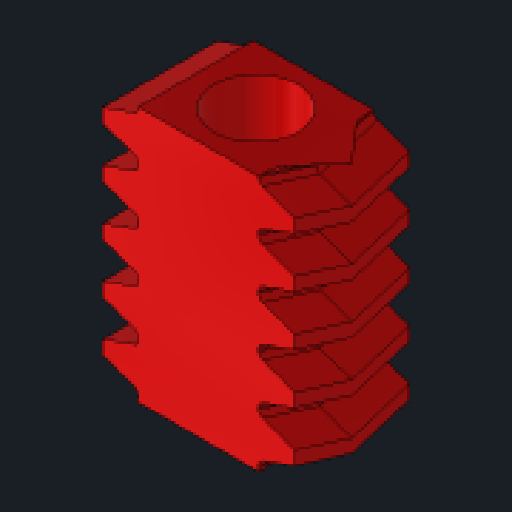
# Autodesk Inventor part: rack
Saved by Autodesk Inventor 2023.2 (Build 272271030, 271C)
## iProperties
Created: 2023-10-23
Part Number: rack
Material: Generic
Document SubType Name: Modeling
Designer: robpl
Density: 1 g/cm^3
Appearance: Red
Author: robpl
## iProperties of the stored document rack_3DPrint.ipt
Created: 2023-10-23
Part Number: rack_3DPrint
Material: Generic
Document SubType Name: Modeling
Designer: robpl
Density: 1 g/cm^3
Appearance: Default
Author: robpl
Autodesk Inventor part; units mm, degrees
ref_plane "YZ Plane" through (0, 0, 0) normal (1, 0, 0) x (0, 1, 0)
sketch "Sketch1" plane through (0, 0, 0) normal (0, 0, 1) x (1, 0, 0)
  line L0 (0, 0) -> (14.5, 0)
  line L1 (14.5, 0) -> (14.5, 20)
  line L2 (14.5, 20) -> (0, 20)
  line L3 (0, 20) -> (0, 0)
  dimension "d0" = 14.5
  dimension "d1" = 20
  constraints: 8 end point, 2 parallel, 1 horizontal, 1 perpendicular
  measures "d0" distance of L2.end L1.end
  measures "d1" distance of L1.end L0.end
extrude "Extrusion1" add sketch "Sketch1" along normal blind 4.5
sketch "Sketch2" plane through (0, 0, 4.5) normal (0, 0, 1) x (1, 0, 0)
  line L0 (14.5, 0) -> (14.5, 20) projected
  line L1 (14.5, 20) -> (0, 20) projected
  line L2 (0, 20) -> (0, 0) projected
  line L3 (0, 0) -> (14.5, 0) projected
  line L4 (14.5, 0) -> (14.5, 20) projected
  line L5 (14.5, 21.4367) -> (11.6875, 20.413)
  line L6 (11.6875, 20.413) -> (11.6875, 19.587)
  line L7 (11.6875, 19.587) -> (14.5, 18.5633)
  line L8 (14.5, 17.5097) -> (11.6875, 16.4861)
  line L9 (11.6875, 16.4861) -> (11.6875, 15.66)
  line L10 (11.6875, 15.66) -> (14.5, 14.6363)
  arc A0 (12, 20.5268) -> (11.6875, 20.0804) centre (12.1625, 20.0804) ccw
  arc A1 (11.6875, 19.9196) -> (12, 19.4732) centre (12.1625, 19.9196) ccw
  line L11 (14.5, 20) -> (0, 20) projected
  arc A2 (11.6875, 15.9926) -> (12, 15.5462) centre (12.1625, 15.9926) ccw
  arc A3 (12, 16.5998) -> (11.6875, 16.1535) centre (12.1625, 16.1535) ccw
  line L12 (14.5, 21.4367) -> (14.5, 18.5633)
  line L13 (7.25, 20) -> (7.25, 0)
  line L14 (0, 0) -> (14.5, 0) projected
  line L15 (0, 21.4367) -> (2.8125, 20.413)
  line L16 (2.8125, 20.413) -> (2.8125, 19.587)
  line L17 (2.8125, 19.587) -> (0, 18.5633)
  arc A4 (2.8125, 20.0804) -> (2.5, 20.5268) centre (2.3375, 20.0804) ccw
  arc A5 (2.5, 19.4732) -> (2.8125, 19.9196) centre (2.3375, 19.9196) ccw
  line L18 (0, 21.4367) -> (0, 18.5633)
  line L19 (0, 17.5097) -> (2.8125, 16.4861)
  line L20 (2.8125, 16.4861) -> (2.8125, 15.66)
  line L21 (2.8125, 15.66) -> (0, 14.6363)
  arc A6 (2.5, 15.5462) -> (2.8125, 15.9926) centre (2.3375, 15.9926) ccw
  arc A7 (2.8125, 16.1535) -> (2.5, 16.5998) centre (2.3375, 16.1535) ccw
  point P0 (11.6875, 20)
  point P1 (13.25, 19.0183)
  point P2 (13.25, 17.0548)
  point P3 (14.5, 18.5633)
  point P4 (11.6875, 20)
  point P5 (14.5, 17.5097)
  point P6 (14.5, 20)
  point P7 (2.8125, 20)
  point P8 (1.25, 19.0183)
  point P9 (0, 20)
  point P10 (1.25, 17.0548)
  dimension "d14" = 70
  dimension "d15" = 3.927
  dimension "d16" = 0.475
  dimension "d17" = 2.8125
  dimension "d18" = 1.25
  dimension "d19" = 1.9635
  constraints: 30 end point, 25 point on line, 23 symmetric about line, 16 point on circle, 8 centre point, 8 tangent, 4 equal length, 3 equal radius, 3 midpoint, 2 vertical, 2 vertical alignment, 1 parallel, 4 other
  measures "d14" angle of L0 L5
  measures "d15" distance of L10.end L7.end
  measures "d16" radius of A0
  measures "d17" distance between parallel lines of L6 L0
  measures "d18" distance from line of L0 point (13.25, 19.018)
  measures "d19" distance of point (13.25, 19.018) point (13.25, 17.055)
ref_plane "Work Plane1" through (13.25, 0, 4.5) normal (1, 0, 0) x (0, 0, -1)
sketch "Sketch3" plane through (14.5, 0, 0) normal (1, 0, 0) x (0, 0, -1)
  line L0 (-4.5, 0) -> (-4.5, 20) projected
  line L1 (-4.5, 20) -> (-4.5, 0) projected
  line L2 (-4.5, 14.6363) -> (0, 13.2175)
  line L3 (0, 0) -> (0, 20) projected
  line L4 (0, 20) -> (-4.5, 20) projected
  dimension "d31" = 17.5
  constraints: 2 end point, 1 point on line
  measures "d31" angle of L4 L2
sweep "Sweep1" cut profiles "Sketch2" path "Sketch3" path curves L2 contours L10 A2 L9 A3 L8 L0 | L7 A1 L6 L1 L0 | L6 A0 L5 L12 L1
pattern_linear "Rectangular Pattern2" count 8 spacing 3.927 along (0, -1, 0) of "Sweep1"
mirror "Mirror2" about plane through (7.25, 10, 0) normal (0, 0, -1)
extrude "Extrusion3" cut sketch "Sketch2" against normal through all contours L2 L19 A7 L20 A6 L21 | L16 A5 L17 L2 L1 | L1 L18 L15 A4 L16
pattern_linear "Rectangular Pattern3" count 10 spacing 3.927 along (0, -1, 0) of "Extrusion3"
sketch "Sketch5" plane through (11.6875, 0, 3.0872) normal (0, -1, 0) x (1, 0, 0)
  line L0 (-8.9697, 1.4128) -> (-8.9697, -7.5872) projected
  line L1 (-8.9697, -7.5872) -> (0.0947, -7.5872) projected
  ellipse E0 centre (0.475, -6.6847) end of major axis (0.475, -5.1782) minor radius 0.475 (0, -6.6847) -> (0.0947, -7.5872) ccw projected
  line L2 (0, -6.1744) -> (0, -6.6847) projected
  ellipse E1 centre (0.475, -6.1744) end of major axis (0.475, -7.6809) minor radius 0.475 (0.3125, -4.7587) -> (0, -6.1744) ccw projected
  line L3 (1.7606, -3.0872) -> (0.3125, -4.7587) projected
  line L4 (1.7606, -3.0872) -> (0.3125, -1.4157) projected
  ellipse E2 centre (0.475, 0) end of major axis (0.475, 1.5065) minor radius 0.475 (0, 0) -> (0.3125, -1.4157) ccw projected
  line L5 (0, 0) -> (0, 0.5103) projected
  ellipse E3 centre (0.475, 0.5103) end of major axis (0.475, -0.9962) minor radius 0.475 (0.0947, 1.4128) -> (0, 0.5103) ccw projected
  line L6 (-8.9697, 1.4128) -> (0.0947, 1.4128) projected
  line L7 (-11.6875, -7.5872) -> (-11.6875, 1.4128) projected
  line L8 (2.8125, 1.4128) -> (2.8125, -3.0872) projected
  point P0 (-11.6875, -3.0872)
  point P1 (-4.1875, -3.0872)
  point P2 (-11.6875, -3.0872)
  dimension "d33" = 0
  dimension "d38" = 14.5
  dimension "d39" = 7.5
  constraints: 1 horizontal alignment, 1 midpoint, 4 other
  measures "d38" distance between parallel lines of L7 L8
  measures "d39" distance from line of point (-4.188, -3.087) L7
hole "Hole1" at (7.5, 0, 0) direction (0, 1, 0) diameter 6.5 end through all
ref_plane "Work Plane2" through (1.25, 17.5097, -4.5) normal (-1, 0, 0) x (0, 0, 1)
equation "\"d19\" = 0.5 * d15"
equation "\"d32\" = 20.5deg"
body "Solid1"
